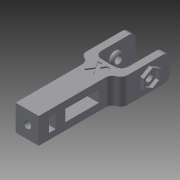
# Autodesk Inventor part: y_tensioner
Saved by Autodesk Inventor 2014 (Build 180170000, 170)
## iProperties
Created: 2016-05-12
Part Number: y_tensioner
Material: Generic
Document SubType Name: Modeling
Designer: 101767
Density: 1 g/cm^3
Appearance: Default
Author: 101767
Autodesk Inventor part; units mm, degrees
ref_plane "XZ Plane" through (0, 0, 0) normal (0, 1, 0) x (-1, 0, 0)
ref_plane "XY Plane" through (0, 0, 0) normal (0, 0, 1) x (1, 0, 0)
sketch "Sketch1" plane through (0, 0, 0) normal (0, 0, 1) x (1, 0, 0)
  line L0 (0, -10.6) -> (0, 63.6) construction
  line L1 (0, 0) -> (-5, 0)
  line L2 (-5, 0) -> (-5, 32)
  line L3 (-5, 32) -> (-8.9, 32)
  line L4 (-8.9, 32) -> (-8.9, 53)
  line L5 (-8.9, 53) -> (-5.9, 53)
  line L6 (-5.9, 35) -> (0, 35)
  line L7 (-13.297, 44) -> (0, 44) construction
  line L8 (-5.9, 53) -> (-5.9, 35)
  line L9 (0, 0) -> (5, 0)
  line L10 (5, 0) -> (5, 32)
  line L11 (5, 32) -> (8.9, 32)
  line L12 (8.9, 32) -> (8.9, 53)
  line L13 (8.9, 53) -> (5.9, 53)
  line L14 (5.9, 35) -> (0, 35)
  line L15 (13.297, 44) -> (0, 44) construction
  line L16 (5.9, 53) -> (5.9, 35)
  dimension "d6" = 32
  dimension "d7" = 3
  dimension "d8" = 3
  dimension "d9" = 5
  dimension "d10" = 18
  dimension "d12" = 9
  dimension "d19" = 5.9
  constraints: 32 end point, 7 symmetric about line, 4 parallel, 4 perpendicular, 3 point on line
  measures "d6" distance of L1.end L2.end
  measures "d7" distance of L4.end L5.end
  measures "d8" distance between parallel lines of L3 L6
  measures "d9" distance of L1.start L1.end
  measures "d10" distance of L5.end L6.start
  measures "d12" distance between parallel lines of L6 L7
  measures "d19" distance between parallel lines of L0 L8
extrude "Extrusion1" add sketch "Sketch1" along normal blind 11.2
ref_plane "Work Plane1" through (4.4, 0, 0) normal (1, 0, 0) x (0, 1, 0)
sketch "Sketch2" plane through (4.4, 0, 0) normal (1, 0, 0) x (0, 1, 0)
  line L0 (35, 0) -> (35, 11.2) construction
  line L1 (53, 0) -> (53, 11.2) construction
  line L2 (35, 5.6) -> (53, 5.6) construction
  circle A0 centre (44, 5.6) radius 2.75
  line L3 (44, -3.8243) -> (44, 13.7141) construction
  line L4 (35, 0) -> (53, 0) construction
  line L5 (53, 11.2) -> (35, 11.2) construction
  point P0 (0, 0)
  dimension "d21" = 5.5
  dimension "d22" = 18
  dimension "d23" = 9
  constraints: 4 end point, 3 midpoint, 1 centre point, 1 perpendicular, 1 point on line
  measures "d21" diameter of A0
  measures "d22" distance between parallel lines of L1 L0
  measures "d23" distance between parallel lines of L0 L3
extrude "Extrusion2" add sketch "Sketch2" along normal up to next
chamfer "Chamfer1" distance 0.5 angle 45 1 edges at (4.4, 41.25, 5.6)
mirror "Mirror1" about plane through (0, 0, 0) normal (1, 0, 0) of "Extrusion2", "Chamfer1"
sketch "Sketch3" plane through (0, 0, 0) normal (1, 0, 0) x (0, 1, 0)
  circle A0 centre (44, 5.6) radius 2.75 construction
  circle A1 centre (44, 5.6) radius 1.65
  point P0 (0, 0)
  dimension "d26" = 3.3
  constraints: 1 centre point, 1 coincident
  measures "d26" diameter of A1
extrude "Extrusion3" cut sketch "Sketch3" along normal through all both and the other way through all
fillet "Fillet1" radius 3 10 edges at (5.9, 35, 5.6) (8.9, 32, 5.6) (-5, 32, 5.6) (5, 32, 5.6) (-8.9, 32, 5.6) (-5.9, 35, 5.6) (-7.4, 53, 11.2) (7.4, 53, 11.2) (7.4, 53, 0) (-7.4, 53, 0)
sketch "Sketch4" plane through (0, 0, 0) normal (1, 0, 0) x (0, 1, 0)
  line L0 (26.0923, 3.1) -> (11.5923, 3.1)
  line L1 (11.5923, 3.1) -> (11.5923, 5.6)
  line L2 (11.5923, 8.1) -> (26.0923, 8.1)
  line L3 (26.0923, 8.1) -> (26.0923, 3.1)
  line L4 (0, 11.2) -> (29, 11.2) construction
  line L5 (29, 0) -> (0, 0) construction
  line L6 (0, 0) -> (0, 11.2) construction
  line L7 (29, 5.6) -> (-2.186, 5.6) construction
  line L8 (11.5923, 5.6) -> (11.5923, 8.1)
  dimension "d33" = 5
  dimension "d34" = 11.2
  dimension "d35" = 5.6
  dimension "d36" = 2.5
  dimension "d37" = 14.5
  constraints: 12 end point, 3 parallel, 3 perpendicular, 1 horizontal, 1 point on line
  measures "d33" distance of L0.end L2.start
  measures "d34" distance between parallel lines of L5 L4
  measures "d35" distance between parallel lines of L5 L7
  measures "d36" distance of L0.end L1.end
  measures "d37" distance of L2.start L2.end
extrude "Extrusion4" cut sketch "Sketch4" along normal through all both and the other way through all
sketch "Sketch5" plane through (5, 0, 11.2) normal (1, 0, 0) x (0, 0, -1)
  line L0 (0, 0) -> (0, 29) construction
  line L1 (11.2, 0) -> (0, 0) construction
  line L2 (11.2, 29) -> (11.2, 0) construction
  line L3 (8.6, 4.5) -> (2.6, 4.5)
  line L4 (2.6, 4.5) -> (2.6, 7.4)
  line L5 (2.6, 7.4) -> (8.6, 7.4)
  line L6 (8.6, 7.4) -> (8.6, 4.5)
  line L7 (5.6, 28.3578) -> (5.6, -4.0028) construction
  dimension "d40" = 6
  dimension "d41" = 2.9
  dimension "d42" = 11.2
  dimension "d43" = 5.6
  dimension "d44" = 3
  dimension "d45" = 4.5
  constraints: 10 end point, 3 parallel, 1 horizontal, 1 perpendicular
  measures "d40" distance of L4.end L5.end
  measures "d41" distance of L5.end L3.start
  measures "d42" distance between parallel lines of L2 L0
  measures "d43" distance between parallel lines of L0 L7
  measures "d44" distance between parallel lines of L4 L7
  measures "d45" distance between parallel lines of L1 L3
extrude "Extrusion5" cut sketch "Sketch5" against normal through all
sketch "Sketch6" plane through (-5, 0, 0) normal (0, -1, 0) x (1, 0, 0)
  line L0 (10, 0) -> (0, 0) construction
  line L1 (0, 0) -> (0, 11.2) construction
  circle A0 centre (5, 5.6) radius 1.65
  point P0 (5, 0)
  dimension "d48" = 3.3
  dimension "d49" = 10
  dimension "d50" = 11.2
  dimension "d51" = 5
  dimension "d52" = 5.6
  constraints: 1 centre point
  measures "d48" diameter of A0
  measures "d49" distance of L0.start L0.end
  measures "d50" distance of L0.end L1.end
  measures "d51" distance from line of A0.centre L1
  measures "d52" distance from line of A0.centre L0
extrude "Extrusion6" cut sketch "Sketch6" against normal up to surface (26.0923 mm away)
sketch "Sketch7" plane through (8.9, 34.6205, 0) normal (1, 0, 0) x (0, 0, -1)
  line L0 (-3, 18.3795) -> (-8.2, 18.3795) construction
  circle A0 centre (-5.6, 9.3795) radius 1.65 construction
  line L1 (-3.9834, 12.1795) -> (-2.3668, 9.3795)
  line L2 (-2.3668, 9.3795) -> (-3.9834, 6.5795)
  line L3 (-3.9834, 6.5795) -> (-7.2166, 6.5795)
  line L4 (-7.2166, 6.5795) -> (-8.8332, 9.3795)
  line L5 (-8.8332, 9.3795) -> (-7.2166, 12.1795)
  line L6 (-7.2166, 12.1795) -> (-3.9834, 12.1795)
  line L7 (-3.4061, 13.1795) -> (-1.2121, 9.3795)
  line L8 (-1.2121, 9.3795) -> (-3.4061, 5.5795)
  line L9 (-3.4061, 5.5795) -> (-7.7939, 5.5795)
  line L10 (-7.7939, 5.5795) -> (-9.9879, 9.3795)
  line L11 (-9.9879, 9.3795) -> (-7.7939, 13.1795)
  line L12 (-7.7939, 13.1795) -> (-3.4061, 13.1795)
  point P0 (0, -34.6205)
  dimension "d55" = 5.6
  dimension "d56" = 1
  constraints: 24 end point, 1 coincident, 1 parallel, 18 other
  measures "d55" distance between parallel lines of L3 L6
  measures "d56" distance between parallel lines of L9 L3
extrude "Extrusion7" add sketch "Sketch7" along normal blind 1.5
sketch "Sketch9" plane through (0, 0, 11.2) normal (0, 0, 1) x (1, 0, 0)
  line L0 (-2.8511, 33.4885) -> (2.9276, 33.4885) construction
  line L1 (2.9276, 33.4885) -> (2.9276, 27.3885) construction
  line L2 (2.9276, 27.3885) -> (-2.8511, 27.3885) construction
  line L3 (-2.8511, 27.3885) -> (-2.8511, 33.4885) construction
  line L4 (2.9424, 27.3885) -> (1.1727, 27.3885)
  line L5 (1.1727, 27.3885) -> (-0.0038, 29.3312)
  line L6 (-0.0038, 29.3312) -> (-1.205, 27.3885)
  line L7 (-1.205, 27.3885) -> (-2.9005, 27.3885)
  line L8 (-2.9005, 27.3885) -> (-0.9183, 30.4583)
  line L9 (-0.9183, 30.4583) -> (-2.8214, 33.4885)
  line L10 (-2.8214, 33.4885) -> (-1.0517, 33.4885)
  line L11 (-1.0517, 33.4885) -> (0.0506, 31.6446)
  line L12 (0.0506, 31.6446) -> (1.1826, 33.4885)
  line L13 (1.1826, 33.4885) -> (2.8782, 33.4885)
  line L14 (2.8782, 33.4885) -> (0.9651, 30.5225)
  line L15 (0.9651, 30.5225) -> (2.9424, 27.3885)
  point P0 (0, 0)
  constraints: 2 other
emboss "Emboss2" sketch "Sketch9" operation cut depth 0.5 direction (0, 0, -1)
equation "\"d23\" = 0.5 * d22"
equation "\"d35\" = 0.5 * d34"
equation "\"d36\" = 0.5 * d33"
equation "\"d43\" = 0.5 * d42"
equation "\"d44\" = 0.5 * d40"
equation "\"d51\" = 0.5 * d49"
equation "\"d52\" = 0.5 * d50"
body "Solid1"
